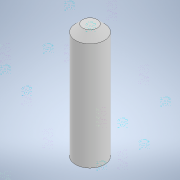
# Autodesk Inventor part: Ch7(5) Part 2 Table Pen
Saved by Autodesk Inventor 2020 (Build 240168000, 168)
## iProperties
Created: 2021-02-25
Part Number: Ch7(5) Part 2 Table Pen
Material: Generic
Document SubType Name: Modeling
Designer: adriggs
Density: 1 g/cm^3
Appearance: Default
Author: adriggs
Autodesk Inventor part; units mm, degrees
ref_plane "YZ Plane" through (0, 0, 0) normal (1, 0, 0) x (0, 1, 0)
ref_plane "XZ Plane" through (0, 0, 0) normal (0, 1, 0) x (-1, 0, 0)
ref_plane "XY Plane" through (0, 0, 0) normal (0, 0, 1) x (1, 0, 0)
sketch "Sketch1" plane through (0, 0, 0) normal (0, 1, 0) x (-1, 0, 0)
  circle A0 centre (0, 0) radius 3.2131
  dimension "d0" = 6.4262
  constraints: 1 centre point, 1 coincident
  measures "d0" diameter of A0
extrude "Extrusion1" add sketch "Sketch1" along normal blind 25.4
chamfer "Chamfer1" distance 1.5875 angle 45 1 edges at (3.2131, 25.4, 0)
body "Solid1"
